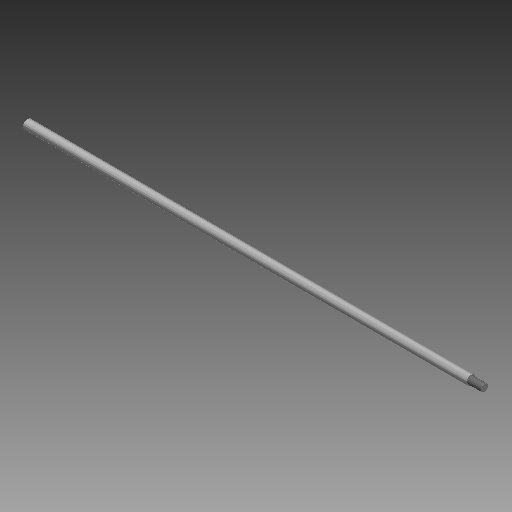
# Autodesk Inventor part: Shaft
Saved by Autodesk Inventor 2019.4 (Build 234330000, 330)
## iProperties
Created: 2020-01-09
Part Number: Shaft
Material: Steel
Document SubType Name: Modeling
Designer: Mark
Mass: 2426.5 g
Surface Area: 638.544 cm^2
Volume: 309.108 cm^3
Density: 7.85 g/cm^3
Appearance: Steel
CustomPartVersion: 1
Length: 1000.000 mm
Author: Mark
Autodesk Inventor part; units mm, degrees
ref_plane "Start Plane" through (0, 0, 0) normal (1, 0, 0) x (0, 1, 0)
ref_plane "XZ Plane" through (0, 0, 0) normal (0, 1, 0) x (-1, 0, 0)
ref_plane "XY Plane" through (0, 0, 0) normal (0, 0, 1) x (1, 0, 0)
sketch "Main Sketch" plane through (0, 0, 0) normal (0, 0, 1) x (1, 0, 0)
  line L0 (0, 0) -> (1000, 0)
  line L1 (0, 4.188) -> (0, 10)
  line L2 (0, 10) -> (970, 10)
  line L3 (970, 10) -> (970, 8)
  line L4 (30, 4.188) -> (30, 0)
  line L5 (0, 4.188) -> (30, 4.188)
  line L6 (30, 0) -> (1000, 0)
  line L7 (1000, 8) -> (1000, 0)
  line L8 (970, 8) -> (1000, 8)
  dimension "d3" = 20
  dimension "d11" = 8.376
  dimension "d32" = 16
  constraints: 18 end point, 4 horizontal, 4 vertical
  measures "d3" diameter of L2 L0
  measures "d11" diameter of L5 L0
  measures "d32" diameter of L8 L0
revolve "Revolution1" add sketch "Main Sketch" angle 360 about axis through (0, 0, 0) along (1, 0, 0)
thread "Thread9" size "M16x2" class "6g" standard "ISO Metric profile" length 30
chamfer "Chamfer6" distance 0.5 angle 45 1 edges at (1000, -8, 0)
thread "Thread12" size "M10x1.5" class "6H" standard "ISO Metric profile" length 30
chamfer "Chamfer8" distance 0.2 angle 45 1 edges at (30, -4.188, 0)
equation "\"Length\" = 1000"
body "Solid1"
